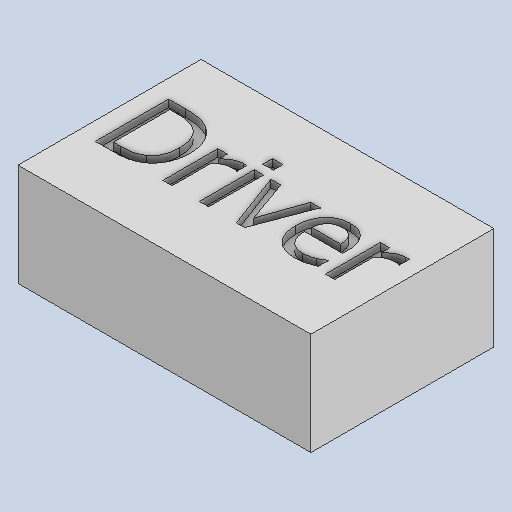
# Autodesk Inventor part: Motor Driver
Saved by Autodesk Inventor 2023 (Build 270158000, 158)
## iProperties
Created: 2022-10-23
Part Number: Motor Driver
Material: Generic
Document SubType Name: Modeling
Designer: chanh
Density: 1 g/cm^3
Appearance: Default
품번: 5
Author: chanh
Autodesk Inventor part; units mm, degrees
ref_plane "YZ Plane" through (0, 0, 0) normal (1, 0, 0) x (0, 1, 0)
ref_plane "XZ Plane" through (0, 0, 0) normal (0, 1, 0) x (-1, 0, 0)
ref_plane "XY Plane" through (0, 0, 0) normal (0, 0, 1) x (1, 0, 0)
sketch "Sketch1" plane through (0, 0, 0) normal (0, 1, 0) x (-1, 0, 0)
  line L0 (20, 12.5) -> (-20, 12.5)
  line L1 (-20, 12.5) -> (-20, -12.5)
  line L2 (-20, -12.5) -> (20, -12.5)
  line L3 (20, -12.5) -> (20, 12.5)
  line L4 (20, 12.5) -> (-20, -12.5) construction
  line L5 (-20, 12.5) -> (20, -12.5) construction
  point P0 (0, 0)
  dimension "d0" = 40
  dimension "d1" = 25
  constraints: 12 end point, 2 midpoint, 2 parallel, 1 horizontal, 1 perpendicular
  measures "d0" distance of L2.end L1.end
  measures "d1" distance of L1.end L0.end
extrude "Extrusion1" add sketch "Sketch1" along normal blind 14
sketch "Sketch2" plane through (0, 14, 0) normal (0, 1, 0) x (1, 0, 0)
  line L0 (-18.5392, 5.6526) -> (18.5392, 5.6526) construction
  line L1 (18.5392, 5.6526) -> (18.5392, -5.6526) construction
  line L2 (18.5392, -5.6526) -> (-18.5392, -5.6526) construction
  line L3 (-18.5392, -5.6526) -> (-18.5392, 5.6526) construction
  line L4 (20, -12.5) -> (20, 12.5) projected
  line L5 (20, 12.5) -> (-20, 12.5) projected
  line L6 (-20, 12.5) -> (-20, -12.5) projected
  line L7 (-20, -12.5) -> (20, -12.5) projected
  spline S0 degree 2 poles (-9.6413, 0.5796) (-9.6413, -0.7899) (-10.7516, -2.9941) (-11.6835, -3.61) knots 0 0 0 1 2 2 2
  spline S1 degree 2 poles (-11.6835, -3.61) (-12.4452, -4.0881) (-14.0093, -4.4123) (-15.2248, -4.4123) knots 0 0 0 1 2 2 2
  line L8 (-15.2248, -4.4123) -> (-17.5263, -4.4123)
  line L9 (-17.5263, -4.4123) -> (-17.5263, 5.5877)
  line L10 (-17.5263, 5.5877) -> (-15.2491, 5.5877)
  spline S2 degree 2 poles (-15.2491, 5.5877) (-13.8391, 5.5877) (-12.2345, 5.1663) (-11.6673, 4.7936) knots 0 0 0 1 2 2 2
  spline S3 degree 2 poles (-11.6673, 4.7936) (-10.7029, 4.1534) (-9.6413, 2.0383) (-9.6413, 0.5796) knots 0 0 0 1 2 2 2
  spline S4 degree 2 poles (-11.0271, 0.5958) (-11.0271, 1.7466) (-11.7888, 3.3754) (-12.5425, 3.8373) knots 0 0 0 1 2 2 2
  spline S5 degree 2 poles (-12.5425, 3.8373) (-13.0773, 4.1534) (-14.2848, 4.437) (-15.1843, 4.437) knots 0 0 0 1 2 2 2
  line L11 (-15.1843, 4.437) -> (-16.1973, 4.437)
  line L12 (-16.1973, 4.437) -> (-16.1973, -3.2615)
  line L13 (-16.1973, -3.2615) -> (-15.1843, -3.2615)
  spline S6 degree 2 poles (-15.1843, -3.2615) (-14.301, -3.2615) (-12.9639, -2.9779) (-12.4209, -2.597) knots 0 0 0 1 2 2 2
  spline S7 degree 2 poles (-12.4209, -2.597) (-11.724, -2.127) (-11.0271, -0.5711) (-11.0271, 0.5958) knots 0 0 0 1 2 2 2
  line L14 (-4.3172, 1.7385) -> (-4.382, 1.7385)
  spline S8 degree 2 poles (-4.382, 1.7385) (-4.5279, 1.779) (-4.8439, 1.7952) (-5.0627, 1.7952) knots 0 0 0 1 2 2 2
  spline S9 degree 2 poles (-5.0627, 1.7952) (-5.5733, 1.7952) (-6.5781, 1.3495) (-7.0319, 0.9119) knots 0 0 0 1 2 2 2
  line L15 (-7.0319, 0.9119) -> (-7.0319, -4.4123)
  line L16 (-7.0319, -4.4123) -> (-8.2961, -4.4123)
  line L17 (-8.2961, -4.4123) -> (-8.2961, 3.0918)
  line L18 (-8.2961, 3.0918) -> (-7.0319, 3.0918)
  line L19 (-7.0319, 3.0918) -> (-7.0319, 1.9735)
  spline S10 degree 2 poles (-7.0319, 1.9735) (-6.3431, 2.5894) (-5.314, 3.0918) (-4.8277, 3.0918) knots 0 0 0 1 2 2 2
  spline S11 degree 2 poles (-4.8277, 3.0918) (-4.6332, 3.0918) (-4.4387, 3.0756) (-4.3172, 3.0513) knots 0 0 0 1 2 2 2
  line L20 (-4.3172, 3.0513) -> (-4.3172, 1.7385)
  line L21 (-2.0481, -4.4123) -> (-3.3123, -4.4123)
  line L22 (-3.3123, -4.4123) -> (-3.3123, 3.0918)
  line L23 (-3.3123, 3.0918) -> (-2.0481, 3.0918)
  line L24 (-2.0481, 3.0918) -> (-2.0481, -4.4123)
  line L25 (-1.959, 4.3398) -> (-3.3934, 4.3398)
  line L26 (-3.3934, 4.3398) -> (-3.3934, 5.6526)
  line L27 (-3.3934, 5.6526) -> (-1.959, 5.6526)
  line L28 (-1.959, 5.6526) -> (-1.959, 4.3398)
  line L29 (5.699, 3.0918) -> (2.8708, -4.4123)
  line L30 (2.8708, -4.4123) -> (1.7363, -4.4123)
  line L31 (1.7363, -4.4123) -> (-1.0676, 3.0918)
  line L32 (-1.0676, 3.0918) -> (0.3019, 3.0918)
  line L33 (0.3019, 3.0918) -> (2.3522, -2.6862)
  line L34 (2.3522, -2.6862) -> (4.3862, 3.0918)
  line L35 (4.3862, 3.0918) -> (5.699, 3.0918)
  spline S12 degree 2 poles (9.913, -4.5824) (8.1139, -4.5824) (6.1366, -2.5646) (6.1366, -0.7008) knots 0 0 0 1 2 2 2
  spline S13 degree 2 poles (6.1366, -0.7008) (6.1366, 1.1307) (8.0572, 3.3025) (9.605, 3.3025) knots 0 0 0 1 2 2 2
  spline S14 degree 2 poles (9.605, 3.3025) (10.3019, 3.3025) (11.3797, 2.8973) (11.7768, 2.4678) knots 0 0 0 1 2 2 2
  spline S15 degree 2 poles (11.7768, 2.4678) (12.182, 2.0383) (12.6115, 0.7984) (12.6115, -0.1011) knots 0 0 0 1 2 2 2
  line L36 (12.6115, -0.1011) -> (12.6115, -0.7899)
  line L37 (12.6115, -0.7899) -> (7.417, -0.7899)
  spline S16 degree 2 poles (7.417, -0.7899) (7.417, -2.0946) (8.7298, -3.4803) (9.8967, -3.4803) knots 0 0 0 1 2 2 2
  spline S17 degree 2 poles (9.8967, -3.4803) (10.31, -3.4803) (11.1123, -3.294) (11.4365, -3.1481) knots 0 0 0 1 2 2 2
  spline S18 degree 2 poles (11.4365, -3.1481) (11.7768, -2.986) (12.2468, -2.7024) (12.4008, -2.5727) knots 0 0 0 1 2 2 2
  line L38 (12.4008, -2.5727) -> (12.4737, -2.5727)
  line L39 (12.4737, -2.5727) -> (12.4737, -3.9504)
  spline S19 degree 2 poles (12.4737, -3.9504) (12.2549, -4.0395) (11.5904, -4.2988) (11.3311, -4.3717) knots 0 0 0 1 2 2 2
  spline S20 degree 2 poles (11.3311, -4.3717) (10.9664, -4.4771) (10.3668, -4.5824) (9.913, -4.5824) knots 0 0 0 1 2 2 2
  spline S21 degree 2 poles (11.3797, 0.1744) (11.3635, 0.685) (11.1528, 1.4305) (10.9502, 1.6817) knots 0 0 0 1 2 2 2
  spline S22 degree 2 poles (10.9502, 1.6817) (10.7314, 1.9654) (10.0426, 2.2652) (9.5321, 2.2652) knots 0 0 0 1 2 2 2
  spline S23 degree 2 poles (9.5321, 2.2652) (9.0296, 2.2652) (8.3246, 1.9654) (8.0329, 1.6736) knots 0 0 0 1 2 2 2
  spline S24 degree 2 poles (8.0329, 1.6736) (7.7493, 1.3738) (7.4575, 0.6526) (7.417, 0.1744) knots 0 0 0 1 2 2 2
  line L40 (7.417, 0.1744) -> (11.3797, 0.1744)
  line L41 (17.8708, 1.7385) -> (17.806, 1.7385)
  spline S25 degree 2 poles (17.806, 1.7385) (17.6601, 1.779) (17.3441, 1.7952) (17.1253, 1.7952) knots 0 0 0 1 2 2 2
  spline S26 degree 2 poles (17.1253, 1.7952) (16.6147, 1.7952) (15.6099, 1.3495) (15.1561, 0.9119) knots 0 0 0 1 2 2 2
  line L42 (15.1561, 0.9119) -> (15.1561, -4.4123)
  line L43 (15.1561, -4.4123) -> (13.8919, -4.4123)
  line L44 (13.8919, -4.4123) -> (13.8919, 3.0918)
  line L45 (13.8919, 3.0918) -> (15.1561, 3.0918)
  line L46 (15.1561, 3.0918) -> (15.1561, 1.9735)
  spline S27 degree 2 poles (15.1561, 1.9735) (15.8449, 2.5894) (16.8741, 3.0918) (17.3603, 3.0918) knots 0 0 0 1 2 2 2
  spline S28 degree 2 poles (17.3603, 3.0918) (17.5548, 3.0918) (17.7493, 3.0756) (17.8708, 3.0513) knots 0 0 0 1 2 2 2
  line L47 (17.8708, 3.0513) -> (17.8708, 1.7385)
  point P0 (0, 0)
  point P1 (-18.5392, 0)
  point P2 (-20, 0)
  point P3 (0, 5.6526)
  point P4 (0, 12.5)
  constraints: 4 midpoint, 1 horizontal alignment, 1 vertical alignment, 2 other
extrude "Extrusion2" cut sketch "Sketch2" against normal blind 1 contours S0 S1 L8 L9 L10 S2 S3 | L14 S8 S9 L15 L16 L17 L18 L19 S10 S11 L20 | L21 L22 L23 L24 | L25 L26 L27 L28 | L29 L30 L31 L32 L33 L34 L35 | S12 S13 S14 S15 L36 L37 S16 S17 S18 L38 L39 S19 S20 | L41 S25 S26 L42 L43 L44 L45 L46 S27 S28 L47
body "Solid1"
